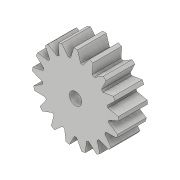
# Autodesk Inventor part: g
Saved by Autodesk Inventor 2019 (Build 230136000, 136)
## iProperties
Created: 2023-07-28
Part Number: g
Material: Generic
Document SubType Name: Modeling
Designer: ahmed
Density: 1 g/cm^3
Appearance: Default
Author: ahmed
## iProperties of the stored document g - Copy - Copy_3DPrint.ipt
Created: 2023-08-01
Part Number: g - Copy - Copy_3DPrint
Material: Generic
Document SubType Name: Modeling
Designer: ahmed
Density: 1 g/cm^3
Appearance: Default
Author: ahmed
Autodesk Inventor part; units mm, degrees
ref_plane "YZ Plane" through (0, 0, 0) normal (1, 0, 0) x (0, 1, 0)
ref_plane "XZ Plane" through (0, 0, 0) normal (0, 1, 0) x (-1, 0, 0)
ref_plane "XY Plane" through (0, 0, 0) normal (0, 0, 1) x (1, 0, 0)
sketch "Sketch4" plane through (0, 0, 0) normal (0, 0, 1) x (1, 0, 0)
  circle A0 centre (0, 0) radius 2.15
  arc A1 (0.6406, 14.9863) -> (-0.6406, 14.9863) centre (0, 0) ccw
  line L0 (-0.6406, 14.9863) -> (-1.724, 11.4276)
  line L1 (0.6406, 14.9863) -> (1.7667, 11.4408)
  arc A2 (-4.8163, 14.2057) -> (-6.0111, 13.7429) centre (0, 0) ccw
  line L2 (-6.0111, 13.7429) -> (-5.7357, 10.0331)
  line L3 (-4.8163, 14.2057) -> (-2.4855, 11.3065)
  arc A3 (-9.6228, 11.5066) -> (-10.5697, 10.6434) centre (0, 0) ccw
  line L4 (-10.5697, 10.6434) -> (-8.9728, 7.2836)
  line L5 (-9.6228, 11.5066) -> (-6.402, 9.6451)
  arc A4 (-13.1296, 7.2535) -> (-13.7008, 6.1065) centre (0, 0) ccw
  line L6 (-13.7008, 6.1065) -> (-10.998, 3.5504)
  line L7 (-13.1296, 7.2535) -> (-9.4539, 6.6811)
  arc A5 (-14.8633, 2.0207) -> (-14.9815, 0.7449) centre (0, 0) ccw
  line L8 (-14.9815, 0.7449) -> (-11.5379, -0.6623)
  line L9 (-14.8633, 2.0207) -> (-11.229, 2.8148)
  arc A6 (-14.5895, -3.485) -> (-14.2389, -4.7174) centre (0, 0) ccw
  line L10 (-14.2389, -4.7174) -> (-10.5195, -4.7855)
  line L11 (-14.5895, -3.485) -> (-11.4876, -1.4317)
  arc A7 (-12.3454, -8.52) -> (-11.5733, -9.5425) centre (0, 0) ccw
  line L12 (-11.5733, -9.5425) -> (-8.0804, -8.2624)
  line L13 (-12.3454, -8.52) -> (-10.1946, -5.4848)
  arc A8 (-8.434, -12.4044) -> (-7.3446, -13.0789) centre (0, 0) ccw
  line L14 (-7.3446, -13.0789) -> (-4.55, -10.6235)
  line L15 (-8.434, -12.4044) -> (-7.5249, -8.7972)
  arc A9 (-3.3835, -14.6134) -> (-2.124, -14.8489) centre (0, 0) ccw
  line L16 (-2.124, -14.8489) -> (-0.4051, -11.5498)
  line L17 (-3.3835, -14.6134) -> (-3.8388, -10.9214)
  arc A10 (2.124, -14.8489) -> (3.3835, -14.6134) centre (0, 0) ccw
  line L18 (3.3835, -14.6134) -> (3.7945, -10.9162)
  line L19 (2.124, -14.8489) -> (0.3656, -11.5707)
  arc A11 (7.3446, -13.0789) -> (8.434, -12.4044) centre (0, 0) ccw
  line L20 (8.434, -12.4044) -> (7.4816, -8.8083)
  line L21 (7.3446, -13.0789) -> (4.5208, -10.6572)
  arc A12 (11.5733, -9.5425) -> (12.3454, -8.52) centre (0, 0) ccw
  line L22 (12.3454, -8.52) -> (10.1583, -5.5109)
  line L23 (11.5733, -9.5425) -> (8.0653, -8.3045)
  arc A13 (14.2389, -4.7174) -> (14.5895, -3.485) centre (0, 0) ccw
  line L24 (14.5895, -3.485) -> (11.4631, -1.4691)
  line L25 (14.2389, -4.7174) -> (10.5206, -4.8302)
  arc A14 (14.9815, 0.7449) -> (14.8633, 2.0207) centre (0, 0) ccw
  line L26 (14.8633, 2.0207) -> (11.2197, 2.7711)
  line L27 (14.9815, 0.7449) -> (11.555, -0.7035)
  arc A15 (13.7008, 6.1065) -> (13.1296, 7.2535) centre (0, 0) ccw
  line L28 (13.1296, 7.2535) -> (9.4611, 6.637)
  line L29 (13.7008, 6.1065) -> (11.0289, 3.5182)
  arc A16 (10.5697, 10.6434) -> (9.6228, 11.5066) centre (0, 0) ccw
  line L30 (9.6228, 11.5066) -> (6.4246, 9.6065)
  line L31 (10.5697, 10.6434) -> (9.0132, 7.2647)
  arc A17 (6.0111, 13.7429) -> (4.8163, 14.2057) centre (0, 0) ccw
  line L32 (4.8163, 14.2057) -> (2.5205, 11.2787)
  line L33 (6.0111, 13.7429) -> (5.7803, 10.0301)
  arc A18 (-1.7177, 11.4483) -> (-2.4855, 11.3065) centre (0, 0) ccw
  arc A19 (2.5339, 11.2957) -> (1.7667, 11.4408) centre (0, 0) ccw
  arc A20 (6.4433, 9.6176) -> (5.7803, 10.0301) centre (0, 0) ccw
  arc A21 (9.4824, 6.6406) -> (9.0132, 7.2647) centre (0, 0) ccw
  arc A22 (11.241, 2.7667) -> (11.0289, 3.5182) centre (0, 0) ccw
  arc A23 (11.4813, -1.4808) -> (11.555, -0.7035) centre (0, 0) ccw
  arc A24 (10.1711, -5.5284) -> (10.5206, -4.8302) centre (0, 0) ccw
  arc A25 (7.4872, -8.8293) -> (8.0653, -8.3045) centre (0, 0) ccw
  arc A26 (3.7921, -10.9377) -> (4.5208, -10.6572) centre (0, 0) ccw
  arc A27 (-0.4152, -11.569) -> (0.3656, -11.5707) centre (0, 0) ccw
  arc A28 (-4.5663, -10.6378) -> (-3.8388, -10.9214) centre (0, 0) ccw
  arc A29 (-8.1008, -8.2699) -> (-7.5249, -8.7972) centre (0, 0) ccw
  arc A30 (-10.5412, -4.7851) -> (-10.1946, -5.4848) centre (0, 0) ccw
  arc A31 (-11.5579, -0.6541) -> (-11.4876, -1.4317) centre (0, 0) ccw
  arc A32 (-11.0137, 3.5653) -> (-11.229, 2.8148) centre (0, 0) ccw
  arc A33 (-5.7373, 10.0547) -> (-6.402, 9.6451) centre (0, 0) ccw
  arc A34 (-8.9821, 7.3032) -> (-9.4539, 6.6811) centre (0, 0) ccw
  point P0 (1.7935, 11.3568)
  point P1 (-1.7943, 11.1967)
  point P2 (-2.4302, 11.2378)
  point P3 (-5.7178, 9.7924)
  point P4 (-6.3257, 9.601)
  point P5 (-8.8692, 7.0656)
  point P6 (-9.3668, 6.6676)
  point P7 (-10.8227, 3.3846)
  point P8 (-11.1429, 2.8337)
  point P9 (-11.3145, -0.7535)
  point P10 (-11.4141, -1.3829)
  point P11 (-10.2782, -4.7899)
  point P12 (-10.1437, -5.4128)
  point P13 (-7.8538, -8.1794)
  point P14 (-7.5034, -8.7116)
  point P15 (-4.3687, -10.4642)
  point P16 (-3.8497, -10.8339)
  point P17 (-0.2936, -11.3357)
  point P18 (0.3239, -11.493)
  point P19 (3.8211, -10.6763)
  point P20 (4.4538, -10.5999)
  point P21 (7.4198, -8.575)
  point P22 (7.9821, -8.2752)
  point P23 (10.0165, -5.3156)
  point P24 (10.4325, -4.8329)
  point P25 (11.2603, -1.3383)
  point P26 (11.4738, -0.7379)
  point P27 (10.9834, 2.8197)
  point P28 (10.9656, 3.4567)
  point P29 (9.2231, 6.597)
  point P30 (8.9764, 7.1845)
  point P31 (6.2172, 9.4833)
  point P32 (5.7749, 9.942)
  point P33 (2.3716, 11.0888)
  dimension "d25" = 4.3
  dimension "d26" = 30
  dimension "d30" = 3.72
  dimension "d31" = 3.72
  dimension "d34" = 360
  constraints: 68 end point, 68 point on circle, 35 centre point, 17 point on line, 3 coincident, 171 other
  measures "d25" diameter of A0
  measures "d26" diameter of A1
  measures "d30" distance of L0.start L0.end
  measures "d31" distance of L1.start L1.end
extrude "Extrusion3" add sketch "Sketch4" along normal blind 10
body "Solid3"
